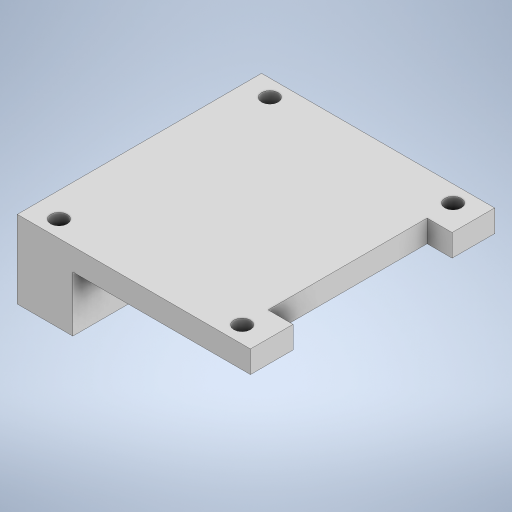
# Autodesk Inventor part: экран кати
Saved by Autodesk Inventor 2024.2 (Build 282272000, 272)
## iProperties
Created: 2026-01-09
Part Number: экран кати
Material: Типовые
Document SubType Name: Modeling
Designer: Service
Density: 1 g/cm^3
Appearance: По умолчанию
Author: Service
Autodesk Inventor part; units mm, degrees
ref_plane "YZ Plane" through (0, 0, 0) normal (1, 0, 0) x (0, 1, 0)
ref_plane "XZ Plane" through (0, 0, 0) normal (0, 1, 0) x (-1, 0, 0)
ref_plane "XY Plane" through (0, 0, 0) normal (0, 0, 1) x (1, 0, 0)
sketch "Эскиз1" plane through (0, 0, 0) normal (0, 1, 0) x (-1, 0, 0)
  line L0 (-16.5, -19) -> (16.5, -19)
  line L1 (16.5, -19) -> (16.5, 19)
  line L2 (16.5, 19) -> (-16.5, 19)
  line L3 (-16.5, 19) -> (-16.5, -19)
  line L4 (-16.5, -19) -> (16.5, 19) construction
  line L5 (16.5, -19) -> (-16.5, 19) construction
  circle A0 centre (16.5, 19) radius 1.5
  circle A1 centre (-16.5, 19) radius 1.5
  circle A2 centre (16.5, -19) radius 1.5
  circle A3 centre (-16.5, -19) radius 1.5
  line L6 (-21, -22) -> (21, -22)
  line L7 (21, -22) -> (21, 22)
  line L8 (21, 22) -> (-21, 22)
  line L9 (-21, 22) -> (-21, -22)
  line L10 (-21, -22) -> (21, 22) construction
  line L11 (21, -22) -> (-21, 22) construction
  line L12 (-21.1405, -14.3289) -> (-16.5, -14.3289)
  line L13 (-16.5, -14.3289) -> (-16.5, 14.3289)
  line L14 (-16.5, 14.3289) -> (-21.1405, 14.3289)
  line L15 (-21.1405, 14.3289) -> (-21.1405, -14.3289)
  line L16 (-21.1405, -14.3289) -> (-16.5, 14.3289) construction
  line L17 (-16.5, -14.3289) -> (-21.1405, 14.3289) construction
  point P0 (0, 0)
  point P1 (-18.8203, 0)
  point P2 (-21, -14.3289)
  point P3 (-21, 14.3289)
  dimension "d0" = 38
  dimension "d1" = 33
  dimension "d2" = 3
  dimension "d3" = 44
  dimension "d4" = 42
  constraints: 36 end point, 6 midpoint, 6 parallel, 4 centre point, 4 coincident, 3 equal radius, 3 horizontal, 3 perpendicular, 1 point on line
  measures "d0" distance of L0.end L1.end
  measures "d1" distance of L1.end L2.end
  measures "d2" diameter of A0
  measures "d3" distance of L6.end L7.end
  measures "d4" distance of L6.start L6.end
extrude "Выдавливание1" add sketch "Эскиз1" along normal blind 4 contours A3 L3 A1 L2 A0 L1 A2 L0 | L0 A2 L1 A0 L2 A1 L3 L14 L9 L8 L7 L6 L12 A3
sketch "Эскиз2" plane through (0, 4, 0) normal (0, 1, 0) x (1, 0, 0)
  line L0 (-21, 22) -> (-21, -22) projected
  line L1 (-21, 22) -> (-11, 22)
  line L2 (-11, 22) -> (-11, 7)
  line L3 (-11, 7) -> (-21, 7)
  line L4 (-21, 7) -> (-21, 22)
  line L5 (-21, -22) -> (21, -22) projected
  line L6 (-21, 7) -> (-11, 7)
  line L7 (-11, 7) -> (-11, -22)
  line L8 (-11, -22) -> (-21, -22)
  line L9 (-21, -22) -> (-21, 7)
  circle A0 centre (-16.5, -19) radius 1.5 projected
  point P0 (0, 0)
  dimension "d7" = 15
  dimension "d8" = 10
  constraints: 16 end point, 4 parallel, 2 horizontal, 2 perpendicular, 1 point on line
  measures "d7" distance of L1.end L2.end
  measures "d8" distance of L2.end L3.end
extrude "Выдавливание2" add sketch "Эскиз2" against normal blind 14 contours L3 L7 L5 L0
